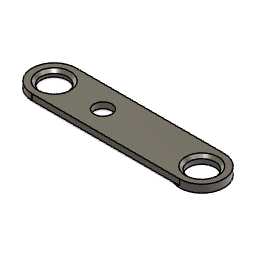
Bielle v2 v2 (Autodesk Fusion 360 design; units mm, degrees)
Autodesk Fusion 360 part; units mm, degrees
sketch "Sketch1" plane through (0, 0, 0) normal (0, 1, 0) x (1, 0, 0)
  line L0 (10.6191, -31.3581) -> (94.7803, -31.3581) construction
  line L1 (17.4831, -11.9367) -> (17.4831, -43.2834) construction
  line L2 (67.4831, -11.9367) -> (67.4831, -43.2834) construction
  circle A0 centre (17.4831, -31.3581) radius 7.5
  circle A1 centre (67.4831, -31.3581) radius 7.5
  line L3 (10.4242, -23.8581) -> (76.5455, -23.8581) construction
  line L4 (7.5967, -38.8581) -> (83.3606, -38.8581) construction
  line L5 (17.4831, -23.8581) -> (67.4831, -23.8581)
  line L6 (17.4831, -38.8581) -> (67.4831, -38.8581)
  circle A2 centre (67.4831, -31.3581) radius 4.5
  circle A3 centre (17.4831, -31.3581) radius 4.5
  line L7 (33.9831, -16.495) -> (33.9831, -43.6658) construction
  circle A4 centre (33.9831, -31.3581) radius 3
  dimension "d1" = 50
  dimension "d2" = 15
  dimension "d3" = 15
  dimension "d4" = 9
  dimension "d5" = 9
  dimension "d9" = 16.5
  dimension "d10" = 6
  constraint horizontal L0
  constraint perpendicular L0 L1
  constraint perpendicular L0 L2
  constraint coincident L0 A0.centre
  constraint coincident L1 A0.centre
  constraint coincident L2 A1.centre
  constraint coincident L0 A1.centre
  constraint horizontal L3
  constraint parallel L3 L4
  constraint tangent A1 L3
  constraint tangent A1 L4
  constraint coincident L1 L5.start
  constraint coincident L3 L5.start
  constraint coincident L3 L5.end
  constraint coincident L2 L5.end
  constraint coincident L1 L6.start
  constraint coincident A0 L6.start
  constraint coincident A1 L6.end
  constraint coincident L2 L6.end
  constraint concentric A1 A2
  constraint concentric A0 A3
  constraint vertical L7
  constraint coincident L0 A4.centre
  constraint coincident L7 A4.centre
  measures "d1" distance of L1 L2
  measures "d2" diameter of A0
  measures "d3" diameter of A1
  measures "d4" diameter of A2
  measures "d5" diameter of A3
  measures "d9" distance of L1 L7
  measures "d10" diameter of A4
extrude "Extrude1" add sketch "Sketch1" along normal blind 2
chamfer "Chamfer1" distance 1 angle 45 2 edges at (13.2876, 2, 29.7308) (63.2876, 2, 29.7308)
sketch "Sketch2" plane through (0, 0, 0) normal (0, -1, 0) x (1, 0, 0)
  circle A0 centre (33.9831, 31.3581) radius 3
  circle A1 centre (17.4831, 31.3581) radius 4.5
  circle A2 centre (67.4831, 31.3581) radius 4.5
  arc A3 (17.4831, 38.8581) -> (17.4831, 23.8581) centre (17.4831, 31.3581) ccw
  line L0 (17.4831, 23.8581) -> (67.4831, 23.8581)
  arc A4 (67.4831, 23.8581) -> (67.4831, 38.8581) centre (67.4831, 31.3581) ccw
  line L1 (67.4831, 38.8581) -> (17.4831, 38.8581)
  circle A5 centre (67.4831, 31.3581) radius 7.5
  circle A6 centre (67.4831, 31.3581) radius 4.5
  constraint concentric A2 A5
  constraint concentric A5 A6
extrude "Extrude2" add sketch "Sketch2" along normal blind 0.6 contours A4 A5
